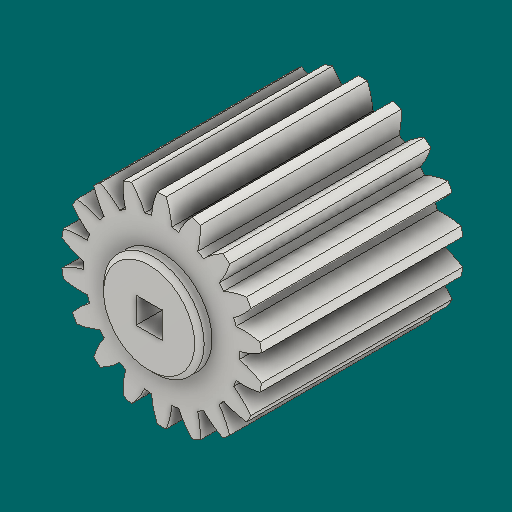
# Autodesk Inventor part: Spur Gear1
Saved by Autodesk Inventor 2023.1 (Build 271208000, 208)
## iProperties
CustomPartVersion: 1
Created: 2022-10-30
Part Number: Spur Gear1
Material: Steel
Document SubType Name: Modeling
Designer: zac-h
Categories: <?xml version="1.0" encoding="UTF-16"?> <MemberInstance><Categories><FamilyTemplate><FamilyTemplateParameter ValueType="xs:double" Id="1" ObjectReferenceKey="da_z" ObjectType="kUserParameterObject"/><FamilyTemplateParameter ValueType="xs:double" Id="2" ObjectReferenceKey="da_b" ObjectType="kUserParameterObject"/><FamilyTemplateParameter ValueType="xs:double" Id="3" ObjectReferenceKey="da_beta" ObjectType="kUserParameterObject"/><FamilyTemplateParameter ValueType="xs:double" Id="4" ObjectReferenceKey="da_da" ObjectType="kUserParameterObject"/><FamilyTemplateParameter ValueType="xs:double" Id="5" ObjectReferenceKey="da_aw" ObjectType="kUserParameterObject"/><FamilyTemplateParameter ValueType="xs:string" Id="6" ObjectReferenceKey="EAIAABAAAAC/AAAAAAAAAIAAAAAAAAAA" ObjectType="83910656" SubObjectId="SurfaceGeometry"/></FamilyTemplate><ParamToTemplateMap><ParamToTemplate CategoryParameter="//CategoryParameter[@InternalName='046C89C9-8512-4d59-83FE-43B91F4F132A']" TemplateParameter="1"/><ParamToTemplate CategoryParameter="//CategoryParameter[@InternalName='2552DF32-E462-4b46-AEBF-C6C7768E72AC']" TemplateParameter="2"/><ParamToTemplate CategoryParameter="//CategoryParameter[@InternalName='C9EE641D-15FC-4fae-A226-E94C4372FDD7']" TemplateParameter="3"/><ParamToTemplate><ParamToTemplate CategoryParameter="//CategoryParameter[@InternalName='00B6519A-459B-49c7-AD84-2E56D39A5744']" ConstantValue="0.000024"/></ParamToTemplate><ParamToTemplate><ParamToTemplate CategoryParameter="//CategoryParameter[@InternalName='04B31F0E-C7A6-4894-AA32-9629BEFACF47']" ConstantValue="1.000000"/></ParamToTemplate><ParamToTemplate><ParamToTemplate CategoryParameter="//CategoryParameter[@InternalName='43CBEC2E-7847-49e7-A936-2F7889FCB2D9']" ConstantValue="0.250000"/></ParamToTemplate><ParamToTemplate><ParamToTemplate CategoryParameter="//CategoryParameter[@InternalName='B1EFC894-105D-4ebd-86BF-FA20ED196853']" ConstantValue="0.333500"/></ParamToTemplate><ParamToTemplate><ParamToTemplate CategoryParameter="//CategoryParameter[@InternalName='51175063-3D10-4879-93E8-6246FE8B403D']" ConstantValue="2061532430.657340"/></ParamToTemplate><ParamToTemplate><ParamToTemplate CategoryParameter="//CategoryParameter[@InternalName='A3A52E27-4454-46a9-B0BD-C932399B70AF']" ConstantValue="0.300000"/></ParamToTemplate><ParamToTemplate><ParamToTemplate CategoryParameter="//CategoryParameter[@InternalName='91B76062-C214-41d9-B1B9-14D2AB99603D']" ConstantValue="0.127000"/></ParamToTemplate><ParamToTemplate><ParamToTemplate CategoryParameter="//CategoryParameter[@InternalName='374E806E-8B8A-4dda-A9AA-1039D6500AD2']" ConstantValue="7.874016"/></ParamToTemplate><ParamToTemplate><ParamToTemplate CategoryParameter="//CategoryParameter[@InternalName='2D373A89-B862-43d6-8D0B-0CBF12AB9F6C']" ConstantValue="0.253073"/></ParamToTemplate><ParamToTemplate CategoryParameter="//CategoryParameter[@InternalName='37777632-D6A2-4fac-9D53-DB8ACD95C989']" TemplateParameter="4"/><ParamToTemplate CategoryParameter="//CategoryParameter[@InternalName='FD1017F1-B727-4f7e-9707-0F86F1FF9423']" TemplateParameter="5"/><ParamToTemplate><ParamToTemplate CategoryParameter="//CategoryParameter[@InternalName='9E1B4470-B2D3-4ff1-B813-535BB4CDF51A']" ConstantValue="3523220.976809"/></ParamToTemplate><ParamToTemplate><ParamToTemplate CategoryParameter="//CategoryParameter[@InternalName='F8452263-BFF6-458c-9FB1-07C4B99E95CD']" ConstantValue="11397033.805607"/></ParamToTemplate><ParamToTemplate><ParamToTemplate CategoryParameter="//CategoryParameter[@InternalName='3E3BB259-FD49-497f-8171-6EBC954A3479']" ConstantValue="2.000000"/></ParamToTemplate><ParamToTemplate CategoryParameter="//CategoryParameter[@InternalName='27C3BAF2-7550-4e4b-AE2C-0DB134B7D9B7']" TemplateParameter="6"/></ParamToTemplateMap><Category DisplayName="Gear" InternalName="DC85795E-93AB-48d5-8EEE-5A27447B64BD" Mnemonic="Gear"><CategoryParameter DisplayName="z" InternalName="046C89C9-8512-4d59-83FE-43B91F4F132A" Mnemonic="z"/><CategoryParameter DisplayName="b" InternalName="2552DF32-E462-4b46-AEBF-C6C7768E72AC" Mnemonic="b"/><CategoryParameter DisplayName="||b|" InternalName="C9EE641D-15FC-4fae-A226-E94C4372FDD7" Mnemonic="beta"/><CategoryParameter DisplayName="x" InternalName="00B6519A-459B-49c7-AD84-2E56D39A5744" Mnemonic="x"/><CategoryParameter DisplayName="a*" InternalName="04B31F0E-C7A6-4894-AA32-9629BEFACF47" Mnemonic="a"/><CategoryParameter DisplayName="c*" InternalName="43CBEC2E-7847-49e7-A936-2F7889FCB2D9" Mnemonic="c"/><CategoryParameter DisplayName="r|.f|*" InternalName="B1EFC894-105D-4ebd-86BF-FA20ED196853" Mnemonic="rf"/><CategoryParameter DisplayName="E" InternalName="51175063-3D10-4879-93E8-6246FE8B403D" Mnemonic="E"/><CategoryParameter DisplayName="||m|" InternalName="A3A52E27-4454-46a9-B0BD-C932399B70AF" Mnemonic="mi"/><Category DisplayName="SpurGear" InternalName="26C5A22E-A91E-4dfd-A3B3-23CCAFAE1764" Mnemonic="SpurGear"><CategoryParameter DisplayName="m" InternalName="91B76062-C214-41d9-B1B9-14D2AB99603D" Mnemonic="m"/><CategoryParameter DisplayName="P" InternalName="374E806E-8B8A-4dda-A9AA-1039D6500AD2" Mnemonic="PP"/><CategoryParameter DisplayName="||a|" InternalName="2D373A89-B862-43d6-8D0B-0CBF12AB9F6C" Mnemonic="alpha"/><CategoryParameter DisplayName="d|.a|" InternalName="37777632-D6A2-4fac-9D53-DB8ACD95C989" Mnemonic="da"/><CategoryParameter DisplayName="a|.w|" InternalName="FD1017F1-B727-4f7e-9707-0F86F1FF9423" Mnemonic="aw"/><CategoryParameter DisplayName="||s||.Flim|" InternalName="9E1B4470-B2D3-4ff1-B813-535BB4CDF51A" Mnemonic="sFlim"/><CategoryParameter DisplayName="||s||.Hlim|" InternalName="F8452263-BFF6-458c-9FB1-07C4B99E95CD" Mnemonic="sHlim"/><CategoryParameter DisplayName="type" InternalName="3E3BB259-FD49-497f-8171-6EBC954A3479" Mnemonic="type"/><CategoryParameter DisplayName="PitchDiameter" InternalName="27C3BAF2-7550-4e4b-AE2C-0DB134B7D9B7" Mnemonic="IDS_PITCHDIAM"/></Category></Category></Categories></MemberInstance>
Density: 1 g/cm^3
Appearance: Steel
d9: 0.000 in
d14: 0.000 in
d15: 0.900 in
d16: 0.000 in
d17: 0.000 in
d18: 0.000 in
d19: 0.900 in
Author: zac-h
Autodesk Inventor part; units mm, degrees
sketch "Sketch1" plane through (0, 0, 0) normal (0, 0, 1) x (1, 0, 0)
  circle A0 centre (0, 0) radius 12.7
  dimension "d0" = 25.4001
  constraints: 1 centre point
  measures "d0" diameter of A0
extrude "Extrusion1" add sketch "Sketch1" along normal blind 25.4
sketch "Sketch2" plane through (0, 0, 0) normal (0, 0, -1) x (-1, 0, 0)
  circle A0 centre (0, 0) radius 12.7 projected
  circle A1 centre (0, 0) radius 11.43
  dimension "d3" = 22.86
  constraints: 1 centre point, 1 coincident
  measures "d3" diameter of A1
surface extrude "Pitch Diameter" sketch "Sketch2" against normal through all shown no curves A1
ref_plane "Work Plane1" through (0, 0, 0) normal (1, 0, 0) x (0, 1, 0)
ref_plane "Work Plane2" through (0, 0, 0) normal (0.9848078, 0.1736482, 0) x (0, 0, 1)
ref_plane "Work Plane3" through (0, 0, 12.7) normal (0, 0, -1) x (-1, 0, 0)
spur gear teeth "Spur Gear" teeth 18 pitch diameter 22.86 tip diameter 25.4001 root diameter 19.6851 face width 25.4 start plane through (0, 0, 0) normal (0, 0, -1) x (-1, 0, 0)
sketch "Sketch3" plane through (0, 0, 25.4) normal (0, 0, 1) x (1, 0, 0)
  line L0 (-1.651, -1.651) -> (1.651, -1.651)
  line L1 (1.651, -1.651) -> (1.651, 1.651)
  line L2 (1.651, 1.651) -> (-1.651, 1.651)
  line L3 (-1.651, 1.651) -> (-1.651, -1.651)
  line L4 (-1.651, -1.651) -> (1.651, 1.651) construction
  line L5 (1.651, -1.651) -> (-1.651, 1.651) construction
  point P0 (0, 0)
  dimension "d20" = 3.302
  dimension "d21" = 3.302
  constraints: 12 end point, 2 midpoint, 2 parallel, 1 horizontal, 1 perpendicular
  measures "d20" distance of L2.end L1.end
  measures "d21" distance of L1.end L0.end
extrude "Extrusion2" cut sketch "Sketch3" against normal through all
sketch "Sketch4" plane through (0, 0, 25.4) normal (0, 0, 1) x (1, 0, 0)
  circle A0 centre (0, 0) radius 6.35
  line L0 (-1.651, 1.651) -> (1.651, 1.651) projected
  line L1 (1.651, 1.651) -> (1.651, -1.651) projected
  line L2 (1.651, -1.651) -> (-1.651, -1.651) projected
  line L3 (-1.651, -1.651) -> (-1.651, 1.651) projected
  arc A1 (-4.8601, 11.7333) -> (-4.5448, 8.7304) centre (5.087, 11.2598) ccw projected
  arc A2 (-4.5448, 8.7304) -> (-5.2884, 8.3011) centre (0, 0) ccw projected
  arc A3 (-5.2884, 8.3011) -> (-7.7313, 10.0756) centre (-12.2948, 1.2244) ccw projected
  arc A4 (-7.7313, 10.0756) -> (-8.58, 9.3634) centre (0, 0) ccw projected
  arc A5 (-8.58, 9.3634) -> (-7.2567, 6.6495) centre (0.9292, 12.3206) ccw projected
  arc A6 (-7.2567, 6.6495) -> (-7.8086, 5.9918) centre (0, 0) ccw projected
  arc A7 (-7.8086, 5.9918) -> (-10.7111, 6.8237) centre (-11.9721, -3.0545) ccw projected
  arc A8 (-10.7111, 6.8237) -> (-11.2651, 5.8642) centre (0, 0) ccw projected
  arc A9 (-11.2651, 5.8642) -> (-9.0933, 3.7666) centre (-3.3408, 11.8954) ccw projected
  arc A10 (-9.0933, 3.7666) -> (-9.387, 2.9597) centre (0, 0) ccw projected
  arc A11 (-9.387, 2.9597) -> (-12.399, 2.7488) centre (-10.2054, -6.965) ccw projected
  arc A12 (-12.399, 2.7488) -> (-12.5914, 1.6577) centre (0, 0) ccw projected
  arc A13 (-12.5914, 1.6577) -> (-9.8332, 0.4293) centre (-7.2078, 10.0354) ccw projected
  arc A14 (-9.8332, 0.4293) -> (-9.8332, -0.4293) centre (0, 0) ccw projected
  arc A15 (-9.8332, -0.4293) -> (-12.5914, -1.6577) centre (-7.2078, -10.0354) ccw projected
  arc A16 (-12.5914, -1.6577) -> (-12.399, -2.7488) centre (0, 0) ccw projected
  arc A17 (-12.399, -2.7488) -> (-9.387, -2.9597) centre (-10.2054, 6.965) ccw projected
  arc A18 (-9.387, -2.9597) -> (-9.0933, -3.7666) centre (0, 0) ccw projected
  arc A19 (-9.0933, -3.7666) -> (-11.2651, -5.8642) centre (-3.3408, -11.8954) ccw projected
  arc A20 (-11.2651, -5.8642) -> (-10.7111, -6.8237) centre (0, 0) ccw projected
  arc A21 (-10.7111, -6.8237) -> (-7.8086, -5.9918) centre (-11.9721, 3.0545) ccw projected
  arc A22 (-7.8086, -5.9918) -> (-7.2567, -6.6495) centre (0, 0) ccw projected
  arc A23 (-7.2567, -6.6495) -> (-8.58, -9.3634) centre (0.9292, -12.3206) ccw projected
  arc A24 (-8.58, -9.3634) -> (-7.7313, -10.0756) centre (0, 0) ccw projected
  arc A25 (-7.7313, -10.0756) -> (-5.2884, -8.3011) centre (-12.2948, -1.2244) ccw projected
  arc A26 (-5.2884, -8.3011) -> (-4.5448, -8.7304) centre (0, 0) ccw projected
  arc A27 (-4.5448, -8.7304) -> (-4.8601, -11.7333) centre (5.087, -11.2598) ccw projected
  arc A28 (-4.8601, -11.7333) -> (-3.819, -12.1122) centre (0, 0) ccw projected
  arc A29 (-3.819, -12.1122) -> (-2.1303, -9.6092) centre (-11.1345, -5.3556) ccw projected
  arc A30 (-2.1303, -9.6092) -> (-1.2847, -9.7583) centre (0, 0) ccw projected
  arc A31 (-1.2847, -9.7583) -> (-0.554, -12.6879) centre (8.6313, -8.8409) ccw projected
  arc A32 (-0.554, -12.6879) -> (0.554, -12.6879) centre (0, 0) ccw projected
  arc A33 (0.554, -12.6879) -> (1.2847, -9.7583) centre (-8.6313, -8.8409) ccw projected
  arc A34 (1.2847, -9.7583) -> (2.1303, -9.6092) centre (0, 0) ccw projected
  arc A35 (2.1303, -9.6092) -> (3.819, -12.1122) centre (11.1345, -5.3556) ccw projected
  arc A36 (3.819, -12.1122) -> (4.8601, -11.7333) centre (0, 0) ccw projected
  arc A37 (4.8601, -11.7333) -> (4.5448, -8.7304) centre (-5.087, -11.2598) ccw projected
  arc A38 (4.5448, -8.7304) -> (5.2884, -8.3011) centre (0, 0) ccw projected
  arc A39 (5.2884, -8.3011) -> (7.7313, -10.0756) centre (12.2948, -1.2244) ccw projected
  arc A40 (7.7313, -10.0756) -> (8.58, -9.3634) centre (0, 0) ccw projected
  arc A41 (8.58, -9.3634) -> (7.2567, -6.6495) centre (-0.9292, -12.3206) ccw projected
  arc A42 (7.2567, -6.6495) -> (7.8086, -5.9918) centre (0, 0) ccw projected
  arc A43 (7.8086, -5.9918) -> (10.7111, -6.8237) centre (11.9721, 3.0545) ccw projected
  arc A44 (10.7111, -6.8237) -> (11.2651, -5.8642) centre (0, 0) ccw projected
  arc A45 (11.2651, -5.8642) -> (9.0933, -3.7666) centre (3.3408, -11.8954) ccw projected
  arc A46 (9.0933, -3.7666) -> (9.387, -2.9597) centre (0, 0) ccw projected
  arc A47 (9.387, -2.9597) -> (12.399, -2.7488) centre (10.2054, 6.965) ccw projected
  arc A48 (12.399, -2.7488) -> (12.5914, -1.6577) centre (0, 0) ccw projected
  arc A49 (12.5914, -1.6577) -> (9.8332, -0.4293) centre (7.2078, -10.0354) ccw projected
  arc A50 (9.8332, -0.4293) -> (9.8332, 0.4293) centre (0, 0) ccw projected
  arc A51 (9.8332, 0.4293) -> (12.5914, 1.6577) centre (7.2078, 10.0354) ccw projected
  arc A52 (12.5914, 1.6577) -> (12.399, 2.7488) centre (0, 0) ccw projected
  arc A53 (12.399, 2.7488) -> (9.387, 2.9597) centre (10.2054, -6.965) ccw projected
  arc A54 (9.387, 2.9597) -> (9.0933, 3.7666) centre (0, 0) ccw projected
  arc A55 (9.0933, 3.7666) -> (11.2651, 5.8642) centre (3.3408, 11.8954) ccw projected
  arc A56 (11.2651, 5.8642) -> (10.7111, 6.8237) centre (0, 0) ccw projected
  arc A57 (10.7111, 6.8237) -> (7.8086, 5.9918) centre (11.9721, -3.0545) ccw projected
  arc A58 (7.8086, 5.9918) -> (7.2567, 6.6495) centre (0, 0) ccw projected
  arc A59 (7.2567, 6.6495) -> (8.58, 9.3634) centre (-0.9292, 12.3206) ccw projected
  arc A60 (8.58, 9.3634) -> (7.7313, 10.0756) centre (0, 0) ccw projected
  arc A61 (7.7313, 10.0756) -> (5.2884, 8.3011) centre (12.2948, 1.2244) ccw projected
  arc A62 (5.2884, 8.3011) -> (4.5448, 8.7304) centre (0, 0) ccw projected
  arc A63 (4.5448, 8.7304) -> (4.8601, 11.7333) centre (-5.087, 11.2598) ccw projected
  arc A64 (4.8601, 11.7333) -> (3.819, 12.1122) centre (0, 0) ccw projected
  arc A65 (3.819, 12.1122) -> (2.1303, 9.6092) centre (11.1345, 5.3556) ccw projected
  arc A66 (2.1303, 9.6092) -> (1.2847, 9.7583) centre (0, 0) ccw projected
  arc A67 (1.2847, 9.7583) -> (0.554, 12.6879) centre (-8.6313, 8.8409) ccw projected
  arc A68 (0.554, 12.6879) -> (-0.554, 12.6879) centre (0, 0) ccw projected
  arc A69 (-0.554, 12.6879) -> (-1.2847, 9.7583) centre (8.6313, 8.8409) ccw projected
  arc A70 (-1.2847, 9.7583) -> (-2.1303, 9.6092) centre (0, 0) ccw projected
  arc A71 (-2.1303, 9.6092) -> (-3.819, 12.1122) centre (-11.1345, 5.3556) ccw projected
  arc A72 (-3.819, 12.1122) -> (-4.8601, 11.7333) centre (0, 0) ccw projected
  dimension "d24" = 12.7
  constraints: 1 centre point, 1 coincident
  measures "d24" diameter of A0
extrude "Extrusion3" add sketch "Sketch4" along normal blind 1.5875 contours A0
chamfer "Chamfer1" distance 0.6 angle 45 1 edges at (-6.35, 0, 26.9875)
sketch "Sketch5" plane through (0, 0, 0) normal (0, 0, -1) x (-1, 0, 0)
  line L0 (3.302, 3.302) -> (-3.302, 3.302)
  line L1 (-3.302, 3.302) -> (-3.302, -3.302)
  line L2 (-3.302, -3.302) -> (3.302, -3.302)
  line L3 (3.302, -3.302) -> (3.302, 3.302)
  line L4 (3.302, 3.302) -> (-3.302, -3.302) construction
  line L5 (-3.302, 3.302) -> (3.302, -3.302) construction
  point P0 (0, 0)
  dimension "d30" = 6.604
  dimension "d31" = 6.604
  constraints: 12 end point, 2 midpoint, 2 parallel, 1 horizontal, 1 perpendicular
  measures "d30" distance of L2.end L1.end
  measures "d31" distance of L1.end L0.end
extrude "Extrusion4" cut sketch "Sketch5" against normal blind 23.8125
chamfer "Chamfer2" distance 1.651 angle 45 4 edges at (0, 3.302, 23.8125) (-3.302, 0, 23.8125) (0, -3.302, 23.8125) (3.302, 0, 23.8125)
equation "\"d0\" = da_da"
equation "\"d1\" = da_b"
equation "\"d3\" = da_d"
equation "\"d15\" = da_aw"
equation "\"d19\" = da_aw"
equation "\"da_da\" = 25.400062"
equation "\"da_b\" = 25.4"
equation "\"da_d\" = 22.86"
equation "\"da_aw\" = 22.86"
body "Solid1"
body "Srf1"
